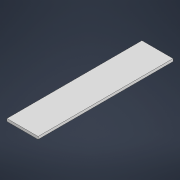
# Autodesk Inventor part: 110033226_ipt_48_船屋梁架
Saved by Autodesk Inventor 2022 (Build 260153000, 153)
## iProperties
Created: 2022-06-28
Part Number: 110033226_ipt_48_船屋梁架
Material: 一般
Document SubType Name: Modeling
Designer: User
Density: 1 g/cm^3
Appearance: 預設
Author: User
Autodesk Inventor part; units mm, degrees
ref_plane "YZ Plane" through (0, 0, 0) normal (1, 0, 0) x (0, 1, 0)
ref_plane "XZ Plane" through (0, 0, 0) normal (0, 1, 0) x (-1, 0, 0)
ref_plane "XY Plane" through (0, 0, 0) normal (0, 0, 1) x (1, 0, 0)
sketch "草圖1" plane through (0, 0, 0) normal (0, 1, 0) x (-1, 0, 0)
  line L0 (0, 0) -> (30, 0)
  line L1 (30, 0) -> (30, -130)
  line L2 (30, -130) -> (0, -130)
  line L3 (0, -130) -> (0, 0)
  dimension "d0" = 30
  dimension "d1" = 130
  constraints: 8 end point, 2 parallel, 1 horizontal, 1 perpendicular
  measures "d0" distance of L1.end L2.end
  measures "d1" distance of L0.end L1.end
extrude "擠出1" add sketch "草圖1" along normal blind 2.5
sketch "草圖3" plane through (0, 0, 0) normal (0, -1, 0) x (1, 0, 0)
  circle A0 centre (-2.5, -2.5) radius 1.7
  line L0 (0, -130) -> (-30, -130) projected
  line L1 (0, 0) -> (0, -130) projected
  line L2 (-30, 0) -> (0, 0) projected
  line L3 (-30, -130) -> (-30, 0) projected
  dimension "d4" = 3.4
  dimension "d5" = 2.5
  dimension "d6" = 2.5
  constraints: 1 centre point
  measures "d4" diameter of A0
  measures "d5" distance from line of L1 A0.centre
  measures "d6" distance from line of L2 A0.centre
extrude "擠出2" cut sketch "草圖3" against normal blind 1.5 contours A0
pattern_linear "矩形陣列1" count 26 spacing 5 along (0, 0, -1) count 6 spacing 5 along (-1, 0, 0) of "擠出2"
